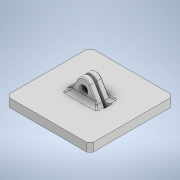
# Autodesk Inventor part: 테스트용 고정판
Saved by Autodesk Inventor 2022 (Build 260153000, 153)
## iProperties
Created: 2022-04-11
Part Number: 테스트용 고정판
Material: 일반
Document SubType Name: Modeling
Designer: USER
Density: 1 g/cm^3
Appearance: 기본값
Author: USER
Autodesk Inventor part; units mm, degrees
ref_plane "YZ Plane" through (0, 0, 0) normal (1, 0, 0) x (0, 1, 0)
ref_plane "XZ Plane" through (0, 0, 0) normal (0, 1, 0) x (-1, 0, 0)
ref_plane "XY Plane" through (0, 0, 0) normal (0, 0, 1) x (1, 0, 0)
sketch "스케치1" plane through (0, 0, 0) normal (0, 0, 1) x (1, 0, 0)
  line L0 (0, 20) -> (17.3205, -10)
  line L1 (17.3205, -10) -> (-17.3205, -10)
  line L2 (-17.3205, -10) -> (0, 20)
  circle A0 centre (0, 0) radius 5
  dimension "d0" = 10
  dimension "d1" = 30
  constraints: 6 end point, 2 coincident, 1 centre point, 1 vertical alignment, 7 other
  measures "d0" diameter of A0
  measures "d1" distance from line of L1 L0.start
extrude "돌출1" add sketch "스케치1" along normal blind 15
sketch "스케치2" plane through (-17.3205, -10, 0) normal (0, -1, 0) x (1, 0, 0)
  line L0 (67.3205, 57.5) -> (-32.6795, 57.5)
  line L1 (-32.6795, 57.5) -> (-32.6795, -42.5)
  line L2 (-32.6795, -42.5) -> (67.3205, -42.5)
  line L3 (67.3205, -42.5) -> (67.3205, 57.5)
  line L4 (0, 0) -> (34.641, 0) projected
  line L5 (34.641, 0) -> (34.641, 15) projected
  point P0 (17.3205, 0)
  point P1 (17.3205, -42.5)
  point P2 (17.3205, 0)
  point P3 (67.3205, 7.5)
  point P4 (34.641, 7.5)
  dimension "d4" = 100
  dimension "d5" = 100
  constraints: 8 end point, 4 midpoint, 2 parallel, 1 horizontal, 1 horizontal alignment, 1 perpendicular, 1 vertical alignment
  measures "d4" distance of L2.end L0.start
  measures "d5" distance of L1.end L2.end
extrude "돌출2" add sketch "스케치2" along normal blind 10
sketch "스케치3" plane through (0, 0, 0) normal (1, 0, 0) x (0, 1, 0)
  line L0 (-10, 0) -> (20, 0) projected
  line L1 (20, 0) -> (20, 15) projected
  line L2 (-10, 15) -> (20, 15) projected
  line L3 (-10, 0) -> (-10, 15) projected
  line L4 (20, 0) -> (20, 15) projected
  line L5 (20, 7.5) -> (-10, 7.5) construction
  line L6 (-10, 57.5) -> (-10, -42.5) projected
  line L7 (20, 6.5) -> (-10, 6.5)
  line L8 (20, 8.5) -> (-10, 8.5)
  point P0 (0, 0)
  point P1 (-10, 8.5)
  point P2 (-10, 6.5)
  dimension "d8" = 1
  dimension "d9" = 1
  constraints: 6 end point, 2 midpoint, 2 parallel
  measures "d8" distance between parallel lines of L5 L7
  measures "d9" distance between parallel lines of L5 L8
extrude "돌출3" cut sketch "스케치3" along normal through all both and the other way through all contours L3 L8 L1 L7
fillet "모깎기1" radius 8 2 edges at (0, 20, 11.75) (0, 20, 3.25)
chamfer "모따기1" distance 0.5 angle 45 6 edges at (12.1244, -1, 6.5) (0, 12, 6.5) (-12.1244, -1, 6.5) (12.1244, -1, 8.5) (0, 12, 8.5) (-12.1244, -1, 8.5)
fillet "모깎기2" radius 5 6 edges at (0, -10, 15) (17.3205, -10, 12) (17.3205, -10, 3) (0, -10, 0) (-17.3205, -10, 12) (-17.3205, -10, 3)
chamfer "모따기2" distance 1 angle 45 14 edges at (10.681, 1.4999, 0) (0, 12, 0) (-10.681, 1.5, 0) (-15.1809, -6.2942, -0.1704) (-17.7073, -9.3301, -2.5) (15.1809, -6.2942, -0.1704) (17.7073, -9.3301, -2.5) (10.681, 1.5, 15) (0, 12, 15) (-10.681, 1.5, 15) (-15.1809, -6.2942, 15.1704) (-17.7073, -9.3301, 17.5) (15.1809, -6.2942, 15.1704) (17.7073, -9.3301, 17.5)
chamfer "모따기3" distance 4 angle 45 4 edges at (50, -15, -42.5) (50, -15, 57.5) (-50, -15, 57.5) (-50, -15, -42.5)
sketch "스케치4" plane through (-17.3205, -10, 0) normal (0, 1, 0) x (1, 0, 0)
  line L0 (34.0637, -6.5) -> (37.5278, -3.5) projected
  line L1 (0.5774, -6.5) -> (34.0637, -6.5) projected
  line L2 (-2.8868, -3.5) -> (0.5774, -6.5) projected
  line L3 (-2.8868, 3.5875) -> (-2.8868, -3.5) projected
  line L4 (-1.4743, 5) -> (-2.8868, 3.5875) projected
  line L5 (36.1153, 5) -> (-1.4743, 5) projected
  line L6 (37.5278, 3.5875) -> (36.1153, 5) projected
  line L7 (37.5278, -3.5) -> (37.5278, 3.5875) projected
  line L8 (37.5278, -11.5) -> (34.0637, -8.5) projected
  line L9 (37.5278, -18.5875) -> (37.5278, -11.5) projected
  line L10 (36.1153, -20) -> (37.5278, -18.5875) projected
  line L11 (-1.4743, -20) -> (36.1153, -20) projected
  line L12 (-2.8868, -18.5875) -> (-1.4743, -20) projected
  line L13 (-2.8868, -11.5) -> (-2.8868, -18.5875) projected
  line L14 (0.5774, -8.5) -> (-2.8868, -11.5) projected
  line L15 (34.0637, -8.5) -> (0.5774, -8.5) projected
  line L16 (-32.6795, 38.5) -> (-28.6795, 42.5) projected
  line L17 (-32.6795, -53.5) -> (-32.6795, 38.5) projected
  line L18 (-28.6795, -57.5) -> (-32.6795, -53.5) projected
  line L19 (63.3205, -57.5) -> (-28.6795, -57.5) projected
  line L20 (67.3205, -53.5) -> (63.3205, -57.5) projected
  line L21 (67.3205, 38.5) -> (67.3205, -53.5) projected
  line L22 (63.3205, 42.5) -> (67.3205, 38.5) projected
  line L23 (-28.6795, 42.5) -> (63.3205, 42.5) projected
  line L24 (34.0637, -6.5) -> (0.5774, -6.5)
  line L25 (0.5774, -6.5) -> (0.5774, -8.5)
  line L26 (0.5774, -8.5) -> (34.0637, -8.5)
  line L27 (34.0637, -8.5) -> (34.0637, -6.5)
  point P0 (17.3205, 0)
  point P1 (0.5774, -8.5)
  dimension "d23" = 33.4863
  constraints: 8 end point, 2 parallel, 1 horizontal, 1 perpendicular, 1 point on line
  measures "d23" distance of L0.start L24.end
extrude "돌출4" cut sketch "스케치4" against normal blind 5 contours L27 L15 L25 L1
chamfer "모따기4" distance 5 angle 45 2 edges at (-16.7432, -10, 7.5) (16.7432, -10, 7.5)
